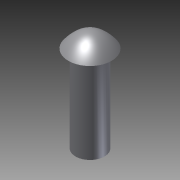
# Autodesk Inventor part: pin
Saved by Autodesk Inventor 2011 SP1 (Build 150282100, 282)
## iProperties
Created: 2013-01-14
Part Number: pin
Document SubType Name: Modeling
Designer: 355283
Density: 1 g/cm^3
Author: 355283
Autodesk Inventor part; units mm, degrees
ref_plane "YZ Plane" through (0, 0, 0) normal (1, 0, 0) x (0, 1, 0)
ref_plane "XZ Plane" through (0, 0, 0) normal (0, 1, 0) x (-1, 0, 0)
ref_plane "XY Plane" through (0, 0, 0) normal (0, 0, 1) x (1, 0, 0)
sketch "Sketch1" plane through (0, 0, 0) normal (0, 0, 1) x (1, 0, 0)
  spline S0 degree 2 poles (-57.6589, -202.4433) (-52.8964, -196.0933) (-48.1339, -196.0933) knots 0 0 0 0.5 0.5 0.5
  line L0 (-57.6589, -202.4433) -> (-54.4839, -202.4433)
  line L1 (-54.4839, -202.4433) -> (-54.4839, -240.5433)
  line L2 (-54.4839, -240.5433) -> (-48.1339, -240.5433)
  line L3 (-48.1339, -240.5433) -> (-48.1339, -196.0933)
  line L4 (-57.6589, -202.4433) -> (-38.6089, -202.4433) construction
  line L5 (-38.6089, -202.4433) -> (-57.6589, -202.4433) construction
  line L6 (-49.7061, -196.0933) -> (-46.5617, -196.0933) construction
  arc A0 (-46.8952, -196.2015) -> (-49.3726, -196.2015) centre (-48.1339, -203.237) ccw construction
  point P0 (0, 0)
  dimension "d0" = 6.35
  dimension "d3" = 6.35
  dimension "d4" = 9.525
  dimension "d5" = 9.525
  dimension "d6" = 38.1
  constraints: 14 end point, 4 perpendicular, 2 horizontal, 2 midpoint, 1 centre point, 1 collinear, 1 point on circle, 3 other
  measures "d0" distance of L1.end L2.end
  measures "d3" distance from line of L0 L3.end
  measures "d4" horizontal distance of L3.end L0.start
  measures "d5" horizontal distance of L4.end L3.end
  measures "d6" distance of L0.end L1.end
revolve "Revolution1" add sketch "Sketch1" angle 360 about axis through (-48.1339, -240.5433, 0) along (0, 1, 0)
equation "\"d5\" = d4"
body "Solid1"
